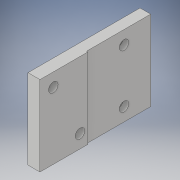
# Autodesk Inventor part: GripperSidePlate
Saved by Autodesk Inventor 2019 (Build 230136000, 136)
## iProperties
Created: 2019-09-28
Part Number: GripperSidePlate
Material: Generic
Document SubType Name: Modeling
Designer: james
Density: 1 g/cm^3
Appearance: Default
Mass: 4.85623 g
Surface Area: 28.9835 cm^2
Volume: 4.85623 cm^3
Author: james
Autodesk Inventor part; units mm, degrees
ref_plane "YZ Plane" through (0, 0, 0) normal (1, 0, 0) x (0, 1, 0)
ref_plane "XZ Plane" through (0, 0, 0) normal (0, 1, 0) x (-1, 0, 0)
ref_plane "XY Plane" through (0, 0, 0) normal (0, 0, 1) x (1, 0, 0)
sketch "Sketch1" plane through (0, 0, 0) normal (1, 0, 0) x (0, 1, 0)
  line L0 (7.5884, 18.4529) -> (-30.5116, 18.4529)
  line L1 (-30.5116, 18.4529) -> (-30.5116, -34.8871)
  line L2 (-30.5116, -34.8871) -> (7.5884, -34.8871)
  line L3 (7.5884, -34.8871) -> (7.5884, 18.4529)
  point P0 (0, 0)
  dimension "d0" = 53.34
  dimension "d1" = 38.1
  constraints: 8 end point, 2 parallel, 1 horizontal, 1 perpendicular
  measures "d0" distance of L2.end L0.start
  measures "d1" distance of L0.start L0.end
extrude "Extrusion1" add sketch "Sketch1" along normal blind 6.35
sketch "Sketch3" plane through (0, 7.5884, 18.4529) normal (0, 1, 0) x (1, 0, 0)
  line L0 (0, 22.86) -> (0.635, 22.86)
  line L1 (0.635, 22.86) -> (0.635, 53.34)
  line L2 (0.635, 53.34) -> (0, 53.34)
  line L3 (0, 53.34) -> (0, 22.86)
  line L4 (5.715, 53.34) -> (6.35, 53.34)
  line L5 (6.35, 53.34) -> (6.35, 22.86)
  line L6 (6.35, 22.86) -> (5.715, 22.86)
  line L7 (5.715, 22.86) -> (5.715, 53.34)
  line L8 (6.35, 53.34) -> (6.35, 0) projected
  line L9 (0, 53.34) -> (0, 0) projected
  line L10 (0, 53.34) -> (6.35, 53.34) projected
  point P0 (0, 18.4529)
  dimension "d19" = 30.48
  dimension "d20" = 30.48
  dimension "d21" = 0
  dimension "d22" = 0
  dimension "d23" = 0.635
  dimension "d24" = 0.635
  dimension "d25" = 0
  constraints: 16 end point, 4 parallel, 2 horizontal, 2 perpendicular, 1 point on line
  measures "d19" distance of L0.end L1.end
  measures "d20" distance of L6.end L4.start
  measures "d21" distance between parallel lines of L8 L5
  measures "d22" distance between parallel lines of L9 L3
  measures "d23" distance of L0.start L0.end
  measures "d24" distance of L5.end L6.end
  measures "d25" distance between parallel lines of L10 L4
extrude "Extrusion2" cut sketch "Sketch3" against normal blind 50.8
sketch "Sketch4" plane through (0, 7.5884, 18.4529) normal (0, 1, 0) x (1, 0, 0)
  line L0 (0.635, 34.7601) -> (-3.8704, 34.7601)
  line L1 (-3.8704, 34.7601) -> (-3.8704, -3.0853)
  line L2 (-3.8704, -3.0853) -> (0.635, -3.0853)
  line L3 (0.635, -3.0853) -> (0.635, 34.7601)
  line L4 (0.635, 53.34) -> (0.635, 22.86) projected
  point P0 (0, 18.4529)
  point P1 (0.635, 53.34)
  dimension "d28" = 0
  constraints: 8 end point, 2 parallel, 1 horizontal, 1 perpendicular
  measures "d28" distance between parallel lines of L3 L4
extrude "Extrusion3" cut sketch "Sketch4" against normal blind 50.8
sketch "Sketch5" plane through (0.635, 7.5884, -34.8871) normal (-1, 0, 0) x (0, 0, 1)
  line L0 (53.34, 0) -> (53.34, -38.1) projected
  line L1 (0, 0) -> (53.34, 0) projected
  line L2 (0, -38.1) -> (0, 0) projected
  point P0 (34.8871, -7.5884)
  point P1 (46.99, -6.35)
  point P2 (34.29, -31.75)
  point P3 (53.34, -38.1)
  point P4 (12.7, -31.75)
  point P5 (12.7, -6.35)
  point P6 (52.07, -25.4)
  point P7 (5.08, 0)
  dimension "d31" = 6.35
  dimension "d32" = 6.35
  dimension "d33" = 31.75
  dimension "d34" = 19.05
  dimension "d35" = 31.75
  dimension "d36" = 12.7
  dimension "d37" = 12.7
  dimension "d38" = 6.35
  constraints: 1 other
  measures "d32" distance from line of L1 point (46.99, -6.35)
  measures "d33" distance from line of L1 point (34.29, -31.75)
  measures "d35" distance from line of L1 point (12.7, -31.75)
  measures "d36" distance from line of L2 point (12.7, -31.75)
  measures "d37" distance from line of L2 point (12.7, -6.35)
  measures "d38" distance from line of L1 point (12.7, -6.35)
hole "Hole2" at (0.635, 1.2384, 12.1029) at (0.635, -24.1616, -0.5971) at (0.635, -24.1616, -22.1871) at (0.635, 1.2384, -22.1871) direction (1, 0, 0) diameter 4.4958 end through all countersink diameter 8.4328 countersink angle 82 clearance for "Flat Head Machine Screw (82)" size "#8" standard "Ansi Unified Screw Threads"
body "Solid1"
